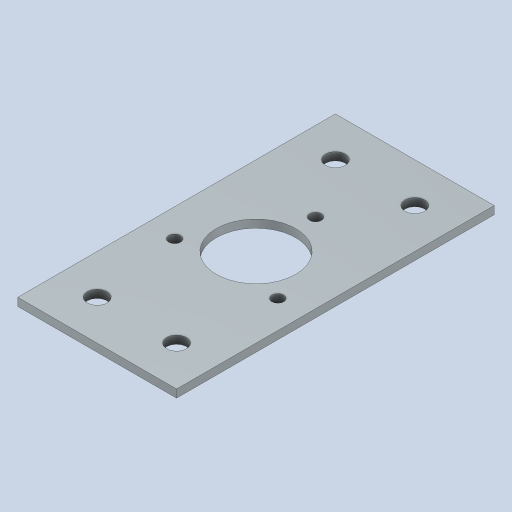
# Autodesk Inventor part: Suporte superior do eixo
Saved by Autodesk Inventor 2023 (Build 270158000, 158)
## iProperties
Created: 2023-03-21
Part Number: Suporte superior do eixo
Material: Zinc
Document SubType Name: Sheet Metal
Designer: Mateus PC
Density: 7 g/cm^3
Sheet Metal Rule: Default_mm
Appearance: Zinc
Mass: 88.5934 g
Surface Area: 137.435 cm^2
Volume: 32.8124 cm^3
Author: Mateus
Autodesk Inventor part; units mm, degrees
ref_plane "YZ Plane" through (0, 0, 0) normal (1, 0, 0) x (0, 1, 0)
ref_plane "XZ Plane" through (0, 0, 0) normal (0, 1, 0) x (-1, 0, 0)
ref_plane "XY Plane" through (0, 0, 0) normal (0, 0, 1) x (1, 0, 0)
sketch "Esboço1" plane through (0, 0, 0) normal (0, 1, 0) x (-1, 0, 0)
  line L0 (0, 0) -> (40, 0)
  line L1 (40, 0) -> (40, -80)
  line L2 (40, -80) -> (0, -80)
  line L3 (0, -80) -> (0, 0)
  circle A0 centre (30, -70) radius 2.5
  circle A1 centre (10, -70) radius 2.5
  circle A2 centre (20, -40) radius 10
  circle A3 centre (30, -10) radius 2.5
  circle A4 centre (10, -10) radius 2.5
  circle A5 centre (20, -55) radius 1.5
  circle A6 centre (32.9904, -32.5) radius 1.5
  circle A7 centre (7.0096, -32.5) radius 1.5
  point P0 (40, -40)
  dimension "d0" = 40
  dimension "d1" = 80
  dimension "d60" = 5
  dimension "d61" = 10
  dimension "d63" = 20
  dimension "d64" = 10
  dimension "d65" = 10
  dimension "d66" = 20
  dimension "d67" = 20
  dimension "d68" = 3
  dimension "d69" = 15
  dimension "d72" = 360
  constraints: 8 centre point, 8 end point, 3 equal radius, 3 horizontal alignment, 3 vertical alignment, 2 parallel, 1 horizontal, 1 midpoint, 1 perpendicular, 7 other
  measures "d0" distance of L1.end L2.end
  measures "d1" distance of L0.end L1.end
  measures "d60" diameter of A0
  measures "d61" distance from line of L1 A0.centre
  measures "d63" distance of A1.centre A0.centre
  measures "d64" distance from line of L2 A0.centre
  measures "d65" distance from line of L0 A3.centre
  measures "d66" distance of point (40, -40) A2.centre
  measures "d67" diameter of A2
  measures "d68" diameter of A5
  measures "d69" distance of A2.centre A5.centre
extrude "Extrusão1" add sketch "Esboço1" along normal blind 2
equation "\"d64\" = d61"
equation "\"d65\" = d64"
equation "\"d66\" = 0.5 * d0"
equation "\"Raio_vergadura\" = Espessura"
equation "\"Largura_alívio_de_vergadura\" = Espessura"
equation "\"Profundidade_alívio_de_vergadura\" = 0.5 * Espessura"
equation "\"Tamanho_alívio_de_dobra\" = 4 * Espessura"
equation "\"Remanescente_mínimo\" = 2 * Espessura"
equation "\"Raiodetransição\" = Raio_vergadura"
equation "\"Tamanho_de_raio_de_Jacobi\" = Raio_vergadura"
equation "\"TamanhoFolga\" = Espessura"
equation "\"Espessura\" = 0.5"
